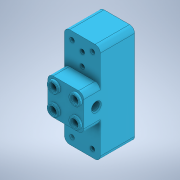
# Autodesk Inventor part: slider
Saved by Autodesk Inventor 2020 (Build 240168000, 168)
## iProperties
Created: 2026-07-07
Part Number: slider
Material: Steel
Document SubType Name: Modeling
Designer: drago
Density: 7.85 g/cm^3
Appearance: Turquoise
Author: drago
Autodesk Inventor part; units mm, degrees
ref_plane "YZ Plane" through (0, 0, 0) normal (1, 0, 0) x (0, 1, 0)
ref_plane "XZ Plane" through (0, 0, 0) normal (0, 1, 0) x (-1, 0, 0)
ref_plane "XY Plane" through (0, 0, 0) normal (0, 0, 1) x (1, 0, 0)
sketch "Sketch1" plane through (0, 0, 0) normal (0, 0, 1) x (1, 0, 0)
  circle A0 centre (4.25, 3.95) radius 1.4
  circle A1 centre (-4.25, 3.95) radius 1.4
  circle A2 centre (-4.25, -3.95) radius 1.4
  circle A3 centre (4.25, -3.95) radius 1.4
  line L0 (-5, 7) -> (5, 7)
  line L1 (7, 5) -> (7, -5)
  line L2 (5, -7) -> (-5, -7)
  line L3 (-7, -5) -> (-7, 5)
  arc A4 (-5, 7) -> (-7, 5) centre (-5, 5) ccw
  arc A5 (7, 5) -> (5, 7) centre (5, 5) ccw
  arc A6 (5, -7) -> (7, -5) centre (5, -5) ccw
  arc A7 (-7, -5) -> (-5, -7) centre (-5, -5) ccw
  circle A8 centre (-4.25, 3.95) radius 2.25
  circle A9 centre (4.25, 3.95) radius 2.25
  circle A10 centre (4.25, -3.95) radius 2.25
  circle A11 centre (-4.25, -3.95) radius 2.25
  point P0 (0, 0)
  constraints: 12 centre point, 8 end point, 8 point on circle, 8 tangent, 3 equal radius, 2 parallel, 1 horizontal, 1 perpendicular
extrude "Extrusion1" add sketch "Sketch1" along normal blind 1 contours A8 | A9 | A10 | A11
extrude "Extrusion2" add sketch "Sketch1" against normal blind 10 contours L0 A5 L1 A6 L2 A7 L3 A4 | A8 | A9 | A10 | A11
sketch "Sketch2" plane through (-7, -5, 0) normal (-1, 0, 0) x (0, 0, 1)
  circle A0 centre (-5, 5) radius 1.45
  point P0 (0, 5)
  constraints: 1 centre point
extrude "Extrusion3" cut sketch "Sketch2" against normal blind 20
chamfer "Chamfer1" distance 0.5 angle 45 2 edges at (-7, 0, -6.45) (7, 0, -6.45)
sketch "Sketch3" plane through (0, 0, -10) normal (0, 0, -1) x (-1, 0, 0)
  circle A0 centre (4.25, -3.95) radius 1.4 projected
  circle A1 centre (-4.25, -3.95) radius 1.4 projected
  circle A2 centre (-4.25, 3.95) radius 1.4 projected
  circle A3 centre (4.25, 3.95) radius 1.4 projected
  point P0 (0, 0)
extrude "Extrusion4" add sketch "Sketch3" against normal blind 6
chamfer "Chamfer2" distance 0.2 angle 45 8 edges at (2.85, -3.95, 1) (-5.65, -3.95, 1) (2.85, 3.95, 1) (-5.65, 3.95, 1) (2, -3.95, 1) (-6.5, -3.95, 1) (-6.5, 3.95, 1) (2, 3.95, 1)
sketch "Sketch4" plane through (-4.25, 3.95, 1) normal (0, 0, 1) x (1, 0, 0)
  circle A0 centre (0, 0) radius 3.95
  circle A1 centre (0, -7.9) radius 3.95
  circle A2 centre (8.5, -7.9) radius 3.95
  circle A3 centre (8.5, 0) radius 3.95
  point P0 (4.25, -3.95)
  point P1 (8.5, -3.95)
  point P2 (0, -3.95)
  constraints: 4 centre point, 2 coincident, 2 equal radius
extrude "Extrusion5" add sketch "Sketch4" along normal blind 4
sketch "Sketch5" plane through (-7, -5, 0) normal (-1, 0, 0) x (0, 0, 1)
  line L0 (-0.5, -2.9) -> (6.5, -2.9)
  line L1 (6.5, -2.9) -> (6.5, 12.9)
  line L2 (6.5, 12.9) -> (-0.5, 12.9)
  line L3 (-0.5, 14.9) -> (8.5, 14.9)
  line L4 (8.5, 14.9) -> (8.5, -4.9)
  line L5 (8.5, -4.9) -> (-0.5, -4.9)
  line L6 (-0.5, 12.9) -> (-0.5, 14.9)
  line L7 (-0.5, -4.9) -> (-0.5, -2.9)
  circle A0 centre (-5, 5) radius 1.45 projected
  circle A1 centre (-5, 5) radius 1.45
  constraints: 16 end point, 3 perpendicular, 2 parallel, 1 centre point, 1 coincident, 1 horizontal, 2 other
sketch "Sketch6" plane through (0, 0, -10) normal (0, 0, -1) x (-1, 0, 0)
  line L0 (7, -1.95) -> (7, 1.95) projected
  line L1 (7, 0) -> (-7, 0)
  line L2 (-7, 0) -> (-7, -17)
  line L3 (-7, -17) -> (7, -17)
  line L4 (7, -17) -> (7, 0)
  line L5 (-5, -7) -> (5, -7) projected
  arc A0 (-7, -5) -> (-5, -7) centre (-5, -5) ccw projected
  arc A1 (5, -7) -> (7, -5) centre (5, -5) ccw projected
  point P0 (0, 0)
  dimension "d37" = 17
  constraints: 8 end point, 2 parallel, 1 horizontal, 1 midpoint, 1 perpendicular
  measures "d37" distance of L2.end L1.end
extrude "Extrusion6" add sketch "Sketch6" against normal blind 8 contours L4 L3 L2 A0 L5 A1
sketch "Sketch7" plane through (0, 0, -2) normal (0, 0, 1) x (1, 0, 0)
  line L0 (-5, -7) -> (5, -7) projected
  line L1 (0, -7) -> (0, -11)
  line L2 (7, 5) -> (7, -17) projected
  line L3 (-7, -17) -> (-7, 5) projected
  line L4 (7, -11) -> (-7, -11)
  line L5 (-7, -11) -> (-7, -17)
  line L6 (-7, -17) -> (7, -17)
  line L7 (7, -17) -> (7, -11)
  point P0 (0, 0)
  constraints: 10 end point, 2 parallel, 1 horizontal, 1 midpoint, 1 perpendicular, 1 point on line, 1 vertical
extrude "Extrusion7" add sketch "Sketch7" along normal blind 12
sketch "Sketch8" plane through (0, 0, -10) normal (0, 0, -1) x (-1, 0, 0)
  arc A0 (-5, 7) -> (-7, 5) centre (-5, 5) ccw projected
  line L0 (7, 5) -> (7, 19.5)
  line L1 (7, 19.5) -> (-7, 19.5)
  line L2 (-7, 19.5) -> (-7, 5)
  arc A1 (7, 5) -> (5, 7) centre (5, 5) ccw projected
  line L3 (5, 7) -> (-5, 7) projected
  point P0 (0, 0)
  constraints: 6 end point, 1 parallel
extrude "Extrusion8" add sketch "Sketch8" against normal blind 3.5
sketch "Sketch9" plane through (0, 0, 10) normal (0, 0, 1) x (1, 0, 0)
  line L0 (7, -11) -> (-7, -11) projected
  line L1 (7, 19.5) -> (7, -17) projected
  line L2 (-7, -11) -> (7, -11)
  line L3 (7, -11) -> (7, -11.4)
  line L4 (7, -11.4) -> (-7, -11.4)
  line L5 (-7, -11.4) -> (-7, -11)
  point P0 (0, 0)
  dimension "d47" = 0.4
  constraints: 8 end point, 2 parallel, 1 horizontal, 1 perpendicular, 1 point on line
  measures "d47" distance of L2.end L3.end
extrude "Extrusion9" cut sketch "Sketch9" against normal up to surface (12 mm away)
sketch "Sketch10" plane through (0, 0, -6.5) normal (0, 0, 1) x (1, 0, 0)
  line L0 (-7, 19.5) -> (7, 19.5) projected
  line L1 (0, 19.5) -> (0, 9.5)
  circle A0 centre (0, 9.5) radius 0.9
  circle A1 centre (0, 14.5) radius 0.9
  point P0 (0, 0)
  dimension "d50" = 10
  dimension "d51" = 1.8
  dimension "d52" = 1.8
  constraints: 2 centre point, 2 end point, 2 midpoint, 1 coincident, 1 vertical
  measures "d50" distance of L1.start L1.end
  measures "d51" diameter of A0
  measures "d52" diameter of A1
extrude "Extrusion10" cut sketch "Sketch10" against normal blind 10
fillet "Fillet1" radius 2 2 edges at (-7, 19.5, -8.25) (7, 19.5, -8.25)
sketch "Sketch12" plane through (0, 0, -10) normal (0, 0, -1) x (-1, 0, 0)
  line L0 (7, -17) -> (-7, -17) projected
  line L1 (7, -17) -> (2, -17)
  line L2 (-7, -17) -> (-2, -17)
  circle A0 centre (4.5, -20) radius 1
  circle A1 centre (4.5, -20) radius 2.5
  circle A2 centre (-4.5, -20) radius 1
  circle A3 centre (-4.5, -20) radius 2.5
  line L3 (7, -17) -> (7, -20)
  line L4 (-7, -17) -> (-7, -20)
  line L5 (-4.5, -22.5) -> (4.5, -22.5)
  point P0 (0, 0)
  dimension "d57" = 5
  constraints: 10 end point, 4 centre point, 4 point on circle, 4 tangent, 2 coincident, 2 point on line
  measures "d57" distance of L0.end L2.end
extrude "Extrusion11" add sketch "Sketch12" against normal blind 3
sketch "Sketch13" plane through (0, 0, 10) normal (0, 0, 1) x (1, 0, 0)
  line L0 (7, -20) -> (7, -17) projected
  line L1 (-7, -17) -> (7, -17) projected
  line L2 (-7, -17) -> (-7, -20) projected
  arc A0 (-7, -20) -> (-4.5, -22.5) centre (-4.5, -20) ccw projected
  line L3 (-4.5, -22.5) -> (4.5, -22.5) projected
  arc A1 (4.5, -22.5) -> (7, -20) centre (4.5, -20) ccw projected
  circle A2 centre (-4.5, -20) radius 1 projected
  circle A3 centre (4.5, -20) radius 1 projected
  line L4 (7, -11.4) -> (-7, -11.4) projected
  line L5 (-7, -11.4) -> (-7, -17) projected
  line L6 (-7, -17) -> (7, -17) projected
  line L7 (7, -17) -> (7, -11.4) projected
  circle A4 centre (4.5, -14.2) radius 0.9
  circle A5 centre (-4.5, -14.2) radius 0.9
  point P0 (0, 0)
  constraints: 2 centre point
extrude "Extrusion12" cut sketch "Sketch13" against normal blind 3 contours L1 L5 L4 L7 | A4 | A5
extrude "Extrusion13" cut sketch "Sketch13" against normal blind 12 contours A4 | A5
fillet "Fillet2" radius 1 1 edges at (0, -11.4, -2)
sketch "Sketch14" plane through (0, 0, -10) normal (0, 0, -1) x (-1, 0, 0)
  circle A0 centre (-4.5, -20) radius 1 projected
  circle A1 centre (4.5, -20) radius 1 projected
  circle A2 centre (0, -27.2111) radius 6.5
  point P0 (0, 0)
  constraints: 1 centre point
extrude "Extrusion14" cut sketch "Sketch14" against normal blind 12 contours A2
fillet "Fillet3" radius 1 2 edges at (-4.4783, -22.5, -8.5) (4.4783, -22.5, -8.5)
sketch "Sketch16" plane through (0, 0, -10) normal (0, 0, -1) x (-1, 0, 0)
  line L0 (-7, -17) -> (7, -17) projected
  line L1 (-7, -17) -> (-1, -17)
  line L2 (-1, -17) -> (-1, -11)
  line L3 (-1, -11) -> (-7, -11)
  line L4 (-7, -11) -> (-7, -17)
  line L5 (-5, 19.5) -> (-0.9, 19.5)
  line L6 (-0.9, 19.5) -> (-0.9, 13)
  line L7 (-0.9, 13) -> (-7, 13)
  line L8 (-7, 13) -> (-7, 17.5)
  line L9 (-7, 17.5) -> (-7, -20) projected
  line L10 (-0.9, 13) -> (-7, 13)
  line L11 (-7, 13) -> (-7, 15)
  line L12 (-7, 15) -> (-0.9, 15)
  line L13 (-0.9, 15) -> (-0.9, 13)
  line L14 (-7, -11) -> (-1, -11)
  line L15 (-1, -11) -> (-1, -13)
  line L16 (-1, -13) -> (-7, -13)
  line L17 (-7, -13) -> (-7, -11)
  circle A0 centre (-3.95, 17.25) radius 0.9
  circle A1 centre (-4, -15) radius 0.9
  arc A2 (-5, 19.5) -> (-7, 17.5) centre (-5, 17.5) ccw projected
  point P0 (0, 0)
  dimension "d83" = 2
  constraints: 32 end point, 8 parallel, 4 horizontal, 4 perpendicular, 2 centre point, 2 point on circle, 2 point on line
  measures "d83" distance of L14.end L15.end
extrude "Extrusion15" cut sketch "Sketch16" against normal blind 6 contours A0 | A1
chamfer "Chamfer3" distance 0.4 angle 45 6 edges at (4.9, -15, -10) (4.85, 17.25, -10) (5.5, -20, -10) (-3.5, -20, -10) (5.5, -20, -7) (-3.5, -20, -7)
sketch "Sketch17" plane through (-4.25, 3.95, 5) normal (0, 0, 1) x (1, 0, 0)
  circle A0 centre (0, 0) radius 3.95 projected
  circle A1 centre (8.5, 0) radius 3.95 projected
  circle A2 centre (8.5, -7.9) radius 3.95 projected
  circle A3 centre (0, -7.9) radius 3.95 projected
  point P0 (4.25, -3.95)
  point P1 (0, -3.95)
  point P2 (8.5, -3.95)
  point P3 (8.5, -3.95)
  point P4 (0, -3.95)
  point P5 (8.5, -3.95)
  point P6 (0, -3.95)
  constraints: 4 other
extrude "Extrusion16" cut sketch "Sketch17" against normal blind 4
sketch "Sketch18" plane through (0, 0, 0) normal (0, 0, 1) x (1, 0, 0)
  line L0 (7, -10.4) -> (-7, -10.4) projected
  line L1 (7, -10.4) -> (7, -5) projected
  arc A0 (5, -7) -> (7, -5) centre (5, -5) ccw projected
  line L2 (-5, -7) -> (5, -7) projected
  arc A1 (-7, -5) -> (-5, -7) centre (-5, -5) ccw projected
  line L3 (-7, -5) -> (-7, -10.4) projected
  line L4 (-7, -10.4) -> (-7, -11.4) projected
  line L5 (-7, -11.4) -> (7, -11.4) projected
  line L6 (7, -11.4) -> (7, -10.4) projected
  line L7 (7, -10.4) -> (-7, -10.4) projected
  circle A2 centre (-4.5, -14.2) radius 0.9 projected
  circle A3 centre (4.5, -14.2) radius 0.9 projected
  line L8 (7, -17) -> (-7, -17) projected
  line L9 (7, -11.4) -> (7, -17) projected
  line L10 (-7, -11.4) -> (7, -11.4) projected
  line L11 (-7, -17) -> (-7, -11.4) projected
  circle A4 centre (4.5, -20) radius 1.4 projected
  arc A5 (4.1777, -22.2315) -> (5.0341, -22.4423) centre (4.8204, -21.4654) ccw projected
  arc A6 (5.0341, -22.4423) -> (7, -20) centre (4.5, -20) ccw projected
  line L12 (7, -20) -> (7, -17) projected
  line L13 (-7, -17) -> (7, -17) projected
  line L14 (-7, -17) -> (-7, -20) projected
  arc A7 (-7, -20) -> (-5.0341, -22.4423) centre (-4.5, -20) ccw projected
  arc A8 (-5.0341, -22.4423) -> (-4.1777, -22.2315) centre (-4.8204, -21.4654) ccw projected
  arc A9 (4.1777, -22.2315) -> (-4.1777, -22.2315) centre (0, -27.2111) ccw projected
  circle A10 centre (-4.5, -20) radius 1.4 projected
  line L15 (-7, -17) -> (-7, -11.4) projected
  line L16 (7, -11.4) -> (7, -17) projected
  point P0 (0, 0)
extrude "Extrusion17" cut sketch "Sketch18" along normal mid plane 30 contours L6 L5 L4 L0 | L0 L3 A1 L2 A0 L1 | L9 L8 L11 L5 | L12 A6 A5 A9 A8 A7 L14 L8 | A2 | A3 | A4 | A10
sketch "Sketch19" plane through (0, 0, -10) normal (0, 0, -1) x (-1, 0, 0)
  arc A0 (5, -7) -> (7, -5) centre (5, -5) ccw projected
  line L0 (7, -5) -> (-7, -5)
  line L1 (-7, -5) -> (-7, -17.5)
  line L2 (-5, -19.5) -> (5, -19.5)
  line L3 (7, -17.5) -> (7, -5)
  arc A1 (5, -19.5) -> (7, -17.5) centre (5, -17.5) ccw
  arc A2 (-7, -17.5) -> (-5, -19.5) centre (-5, -17.5) ccw
  point P0 (0, 0)
  dimension "d98" = 2
  constraints: 8 end point, 4 point on circle, 4 tangent, 2 centre point, 2 parallel, 1 equal radius, 1 horizontal, 1 perpendicular
  measures "d98" radius of A1
extrude "Extrusion18" add sketch "Sketch19" against normal up to surface (3.5 mm away)
sketch "Sketch20" plane through (0, 0, -10) normal (0, 0, -1) x (-1, 0, 0)
  circle A0 centre (-3.95, 17.25) radius 1.3 projected
  circle A1 centre (-3.95, 17.25) radius 1.3
  point P0 (0, 0)
  constraints: 1 centre point, 1 coincident
extrude "Extrusion19" add sketch "Sketch20" against normal blind 3.5
sketch "Sketch21" plane through (0, 0, -10) normal (0, 0, -1) x (-1, 0, 0)
  arc A0 (-5, 19.5) -> (-7, 17.5) centre (-5, 17.5) ccw projected
  arc A1 (5, -19.5) -> (7, -17.5) centre (5, -17.5) ccw projected
  circle A2 centre (-4, -16.5) radius 0.9
  circle A3 centre (4, -16.5) radius 0.9
  circle A4 centre (4, 16.5) radius 0.9
  circle A5 centre (-4, 16.5) radius 0.9
  constraints: 4 centre point
extrude "Extrusion20" cut sketch "Sketch21" against normal blind 3.5
sketch "Sketch22" plane through (-7, -5, 0) normal (-1, 0, 0) x (0, 0, 1)
  circle A0 centre (-5, 5) radius 1.45 projected
  circle A1 centre (-5, 5) radius 1.525
  point P0 (0, 5)
  dimension "d110" = 3.05
  constraints: 1 centre point, 1 coincident
  measures "d110" diameter of A1
extrude "Extrusion21" cut sketch "Sketch22" against normal blind 20
sketch "Sketch23" plane through (0, 0, -10) normal (0, 0, -1) x (-1, 0, 0)
  circle A0 centre (-4, -16.5) radius 0.9 projected
  circle A1 centre (4, 16.5) radius 0.9 projected
  circle A2 centre (4, -16.5) radius 0.9 projected
  circle A3 centre (-4, 16.5) radius 0.9 projected
  line L0 (7, -17.5) -> (7, 17.5) projected
  arc A4 (7, 17.5) -> (5, 19.5) centre (5, 17.5) ccw projected
  line L1 (5, 19.5) -> (-5, 19.5) projected
  arc A5 (-5, 19.5) -> (-7, 17.5) centre (-5, 17.5) ccw projected
  line L2 (-7, 17.5) -> (-7, -17.5) projected
  arc A6 (-7, -17.5) -> (-5, -19.5) centre (-5, -17.5) ccw projected
  line L3 (-5, -19.5) -> (5, -19.5) projected
  arc A7 (5, -19.5) -> (7, -17.5) centre (5, -17.5) ccw projected
  circle A8 centre (0, 14.5) radius 0.9 projected
  circle A9 centre (0, 9.5) radius 0.9 projected
  point P0 (0, 0)
extrude "Extrusion22" add sketch "Sketch23" along normal blind 10
body "Solid1"
